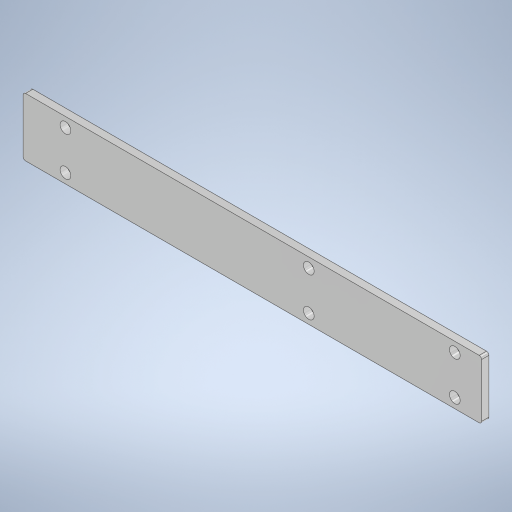
# Autodesk Inventor part: slider_plate
Saved by Autodesk Inventor 2024 (Build 280153000, 153)
## iProperties
Created: 2025-06-12
Part Number: slider_plate
Material: アルミニウム
Document SubType Name: Modeling
Designer: 1412z
Density: 2.7 g/cm^3
Appearance: アルミニウム - つや出し
Author: 1412z
Autodesk Inventor part; units mm, degrees
ref_plane "YZ Plane" through (0, 0, 0) normal (1, 0, 0) x (0, 1, 0)
ref_plane "XZ Plane" through (0, 0, 0) normal (0, 1, 0) x (-1, 0, 0)
ref_plane "XY Plane" through (0, 0, 0) normal (0, 0, 1) x (1, 0, 0)
sketch "スケッチ1" plane through (0, 0, 0) normal (0, 0, 1) x (1, 0, 0)
  line L0 (0, 0) -> (-94.2, 0)
  line L1 (-94.2, 0) -> (-94.2, -12)
  line L2 (-94.2, -12) -> (0, -12)
  line L3 (0, -12) -> (0, 0)
  circle A0 centre (-85.5, -2) radius 1.1
  circle A1 centre (-85.5, -10) radius 1.1
  circle A2 centre (-35.5, -10) radius 1.1
  circle A3 centre (-35.5, -2) radius 1.1
  circle A4 centre (-5.5, -2) radius 1.1
  circle A5 centre (-5.5, -10) radius 1.1
  dimension "d0" = 94.2
  dimension "d1" = 12
  dimension "d2" = 2.2
  dimension "d3" = 2.2
  dimension "d4" = 8.7
  dimension "d5" = 2.2
  dimension "d7" = 2.2
  dimension "d8" = 2.2
  dimension "d9" = 50
  dimension "d10" = 50
  dimension "d11" = 30
  dimension "d12" = 2.2
  dimension "d13" = 30
  constraints: 8 end point, 6 centre point, 2 parallel, 1 horizontal, 1 perpendicular
  measures "d0" distance of L2.end L1.end
  measures "d1" distance of L1.end L0.end
  measures "d2" diameter of A0
  measures "d3" diameter of A1
  measures "d4" distance from line of L1 A1.centre
  measures "d5" diameter of A2
  measures "d7" diameter of A3
  measures "d8" diameter of A4
  measures "d9" distance of A1.centre A2.centre
  measures "d10" distance of A0.centre A3.centre
  measures "d11" distance of A4.centre A3.centre
  measures "d12" diameter of A5
  measures "d13" distance of A2.centre A5.centre
extrude "押し出し1" add sketch "スケッチ1" along normal blind 1.5
fillet "フィレット1" radius 0.5 4 edges at (0, 0, 0.75) (0, -12, 0.75) (-94.2, 0, 0.75) (-94.2, -12, 0.75)
